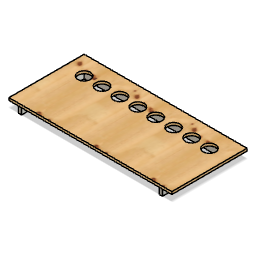
Organ (Autodesk Fusion 360 archive; units mm, degrees)
design "Table"
Autodesk Fusion 360 part; units mm, degrees
sketch "Sketch1" plane through (0, 0, 0) normal (0, 1, 0) x (1, 0, 0)
  line L0 (650, 300) -> (-650, 300)
  line L1 (-650, 300) -> (-650, -300)
  line L2 (-650, -300) -> (650, -300)
  line L3 (650, -300) -> (650, 300)
  line L4 (650, 300) -> (-650, -300) construction
  line L5 (-650, 300) -> (650, -300) construction
  line L6 (0, 0) -> (650, 0)
  line L7 (0, 0) -> (0, 300)
  line L8 (0, 0) -> (0, -300)
  line L9 (0, 0) -> (-650, 0)
  circle A0 centre (-500, 150) radius 50
  circle A1 centre (-357.1429, 150) radius 50
  circle A2 centre (-214.2857, 150) radius 50
  circle A3 centre (-71.4286, 150) radius 50
  circle A4 centre (71.4286, 150) radius 50
  circle A5 centre (214.2857, 150) radius 50
  circle A6 centre (357.1429, 150) radius 50
  circle A7 centre (500, 150) radius 50
  dimension "d1" = 1300
  dimension "d2" = 600
  dimension "d3" = 100
  dimension "d5" = 150
  dimension "d7" = 150
  dimension "d10" = 1000
  dimension "d11" = 0
  constraint horizontal L0
  constraint perpendicular L0 L1
  constraint parallel L0 L2
  constraint parallel L1 L3
  constraint coincident L4 L6.start
  constraint coincident L5 L6.start
  constraint coincident L6.start L7.start
  constraint midpoint L3 L6.end
  constraint midpoint L0 L7.end
  constraint midpoint L2 L8.end
  constraint midpoint L1 L9.end
  measures "d1" distance of L1.end L2.end
  measures "d2" distance of L0.end L1.end
  measures "d3" diameter of A0
  measures "d5" distance of L0 A0.centre
  measures "d7" distance of L1 A0.centre
extrude "Extrude1" add sketch "Sketch1" along normal blind 20 makes body 1
sketch "Sketch2" plane through (0, 0, 0) normal (0, -1, 0) x (1, 0, 0)
  circle A0 centre (214.2857, -150) radius 50
  circle A1 centre (71.4286, -150) radius 50
  circle A2 centre (-71.4286, -150) radius 50
  circle A3 centre (-357.1429, -150) radius 50
  circle A4 centre (-214.2857, -150) radius 50
  circle A5 centre (-500, -150) radius 50
  circle A6 centre (357.1429, -150) radius 50
  circle A7 centre (500, -150) radius 50
  line L0 (650, -300) -> (650, 300)
  line L1 (650, 300) -> (-650, 300)
  line L2 (-650, 300) -> (-650, -300)
  line L3 (-650, -300) -> (650, -300)
  line L4 (-575, 300) -> (-550, 300)
  line L5 (-550, 300) -> (-550, -225)
  line L6 (-550, -225) -> (-575, -225)
  line L7 (-575, -225) -> (-575, 300)
  line L8 (575, 300) -> (550, 300)
  line L9 (550, 300) -> (550, -225)
  line L10 (550, -225) -> (575, -225)
  line L11 (575, -225) -> (575, 300)
  line L12 (-550, -225) -> (550, -225)
  line L13 (550, -225) -> (550, -200)
  line L14 (550, -200) -> (-550, -200)
  line L15 (-550, -200) -> (-550, -225)
  dimension "d14" = 25
  dimension "d15" = 25
  dimension "d16" = 100
  dimension "d17" = 100
  dimension "d18" = 25
  dimension "d19" = 100
  constraint horizontal L4
  constraint vertical L5
  constraint horizontal L6
  constraint vertical L7
  constraint coincident L1 L4.start
  constraint horizontal L8
  constraint vertical L9
  constraint horizontal L10
  constraint vertical L11
  constraint coincident L1 L8.start
  constraint horizontal L12
  constraint vertical L13
  constraint horizontal L14
  constraint vertical L15
  constraint coincident L9 L13.end
  constraint coincident L9.end L10.start
  measures "d14" distance of L4.start L4.end
  measures "d15" distance of L8.start L8.end
  measures "d16" distance of L2 L5
  measures "d17" distance of L0 L9
  measures "d18" distance of L5.end L14.end
  measures "d19" distance of L3 L14
extrude "Extrude2" add sketch "Sketch2" along normal blind 50 separate body contours L5 L9 L12 L13 L14 L15 | L1 L8 L9 L10 L11 L13 | L1 L4 L5 L6 L7 L15 makes body 2
equation "d3 = pipeDiameter"
equation "pipeDiameter = 100 mm"
equation "d5 = margin + pipeDiameter / 2"
equation "margin = 100 mm"
equation "d7 = margin + pipeDiameter / 2"
equation "d10 = 1300 mm - margin * 2 - pipeDiameter"
equation "d16 = margin"
equation "d17 = margin"
equation "d19 = margin"

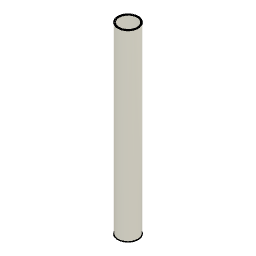
design "Pipe MM"
Autodesk Fusion 360 part; units mm, degrees
sketch "Sketch1" plane through (0, 0, 0) normal (0, 1, 0) x (1, 0, 0)
  circle A0 centre (0, 0) radius 50
  circle A1 centre (0, 0) radius 55
  dimension "d1" = 100
  dimension "d2" = 110
  constraint coincident A0.centre A1.centre
  measures "d1" diameter of A0
  measures "d2" diameter of A1
extrude "Extrude1" add sketch "Sketch1" along normal blind 1000
equation "d2 = d1 + 10 mm"
